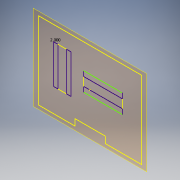
# Autodesk Inventor part: RetroTape
Saved by Autodesk Inventor 2018 (Build 220112000, 112)
## iProperties
Created: 2017-09-17
Part Number: RetroTape
Material: Generic
Document SubType Name: Modeling
Designer: Techbrick Alt
Density: 1 g/cm^3
Appearance: PTFE
Author: Techbrick Alt
Autodesk Inventor part; units mm, degrees
ref_plane "YZ Plane" through (0, 0, 0) normal (1, 0, 0) x (0, 1, 0)
ref_plane "XZ Plane" through (0, 0, 0) normal (0, 1, 0) x (-1, 0, 0)
ref_plane "XY Plane" through (0, 0, 0) normal (0, 0, 1) x (1, 0, 0)
ref_plane "Work Plane1" through (0, 0, 0) normal (0, 0, 1) x (1, 0, 0)
sketch "Sketch3" plane through (0, 0, 0) normal (0, 0, 1) x (1, 0, 0)
  line L0 (-431.8, 279.4) -> (-381, 279.4)
  line L1 (-381, 279.4) -> (-381, -177.8)
  line L2 (-381, -177.8) -> (-431.8, -177.8)
  line L3 (-431.8, -177.8) -> (-431.8, 279.4)
  line L4 (-279.4, 279.4) -> (-228.6, 279.4)
  line L5 (-228.6, 279.4) -> (-228.6, -177.8)
  line L6 (-228.6, -177.8) -> (-279.4, -177.8)
  line L7 (-279.4, -177.8) -> (-279.4, 279.4)
  line L8 (-76.2, 161.2348) -> (381, 161.2348)
  line L9 (381, 161.2348) -> (381, 101.6)
  line L10 (381, 101.6) -> (-76.2, 101.6)
  line L11 (-76.2, 101.6) -> (-76.2, 161.2348)
  line L12 (-76.2, 0) -> (381, 0)
  line L13 (381, 0) -> (381, -59.6348)
  line L14 (381, -59.6348) -> (-76.2, -59.6348)
  line L15 (-76.2, -59.6348) -> (-76.2, 0)
  line L16 (-177.8, -457.2) -> (-177.8, -381) projected
  line L17 (-177.8, -381) -> (177.8, -381) projected
  line L18 (177.8, -381) -> (177.8, -457.2) projected
  line L19 (177.8, -457.2) -> (609.6, -457.2) projected
  line L20 (609.6, -457.2) -> (609.6, 457.2) projected
  line L21 (609.6, 457.2) -> (-609.6, 457.2) projected
  line L22 (-609.6, 457.2) -> (-609.6, -457.2) projected
  line L23 (-609.6, -457.2) -> (-177.8, -457.2) projected
  line L24 (-279.4, -177.8) -> (-381, -177.8) projected
  line L25 (-381, -177.8) -> (-381, 279.4) projected
  line L26 (-381, 279.4) -> (-279.4, 279.4) projected
  line L27 (-279.4, 279.4) -> (-279.4, -177.8) projected
  line L28 (381, 101.6) -> (381, 0) projected
  line L29 (381, 0) -> (-76.2, 0) projected
  line L30 (-76.2, 0) -> (-76.2, 101.6) projected
  line L31 (-76.2, 101.6) -> (381, 101.6) projected
  point P0 (0, 0)
  dimension "d4" = 50.8
  constraints: 32 end point, 14 collinear, 8 parallel, 4 horizontal, 4 perpendicular
  measures "d4" distance of L0.start L0.end
extrude "Extrusion2" add sketch "Sketch3" along normal blind 2.54 contours L0 L1 L2 L3 | L4 L5 L6 L7 | L8 L9 L10 L11 | L12 L13 L14 L15
body "Solid2"
